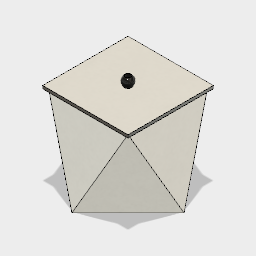
Nagomi v11 (Autodesk Fusion 360 design; units mm, degrees)
Autodesk Fusion 360 part; units mm, degrees
sketch "Sketch1" plane through (0, 0, 0) normal (0, 1, 0) x (1, 0, 0)
  line L0 (40, -40) -> (-40, -40)
  line L1 (-40, -40) -> (-40, 40)
  line L2 (-40, 40) -> (40, 40)
  line L3 (40, 40) -> (40, -40)
  line L4 (40, -40) -> (-40, 40) construction
  line L5 (-40, -40) -> (40, 40) construction
  dimension "d1" = 80
  dimension "d2" = 80
  measures "d1" distance of L1.end L2.end
  measures "d2" distance of L0.end L1.end
extrude "Extrude1" add sketch "Sketch1" along normal blind 80 draft 11.7 makes body 1
ref_plane "WorkPlane1" through (0, 80, 0) normal (0, 1, 0) x (1, 0, 0)
mirror "Mirror1" about plane through (0, 80, 0) normal (0, 1, 0) of bodies 1 makes body 2
move_body "Move1" bodies 2 to x (0.707107, 0, -0.707107) y (0, 1, 0) z (0.707107, 0, 0.707107) at (0, 0, 0)
move_body "Move2" bodies 2 to x (1, 0, 0) y (0, 1, 0) z (0, 0, 1) at (0, -80, 0)
combine "Combine1" operation intersect target body 1 tool bodies 2
shell "Shell1" thickness 2 removed faces 1 at (-18.8557, 80, 0.0004) on bodies 1
move_body "Move3" bodies 1 to x (0.707107, 0, -0.707107) y (0, 1, 0) z (0.707107, 0, 0.707107) at (0, 0, 0)
ref_plane "WorkPlane3" through (0, 75.2, 0) normal (0, 1, 0) x (0.707107, 0, -0.707107)
sketch "Sketch5" plane through (0, 75.2, 0) normal (0, 1, 0) x (1, 0, 0)
  line L0 (-37.9576, 37.9576) -> (37.9576, 37.9576)
  line L1 (37.9576, 37.9576) -> (37.9576, -37.9576)
  line L2 (37.9576, -37.9576) -> (-37.9576, -37.9576)
  line L3 (-37.9576, -37.9576) -> (-37.9576, 37.9576)
  point P0 (-37.9576, 37.9576)
  point P1 (37.9576, -37.9576)
extrude "Extrude2" add sketch "Sketch5" along normal blind 4.8 separate body makes body 3
ref_plane "WorkPlane4" through (0, 80, 0) normal (0, 1, 0) x (0, 0, 1)
sketch "Sketch6" plane through (0, 80, 0) normal (0, 1, 0) x (1, 0, 0)
  line L0 (-40, -39.9981) -> (-40, 39.9981)
  line L1 (-40, -37.8323) -> (-43, -37.8323) construction
  line L2 (39.9981, -40) -> (-39.9981, -40)
  line L3 (-36.5496, -40) -> (-36.5496, -43) construction
  line L4 (-36.5496, -43) -> (-44, -43)
  line L5 (-43, -37.8323) -> (-43, -43)
  line L6 (-39.9981, 40) -> (39.9981, 40)
  line L7 (35.8022, 40) -> (35.8022, 43) construction
  line L8 (40, 39.9981) -> (40, -39.9981)
  line L9 (40, 37.0082) -> (43, 37.0082) construction
  line L10 (43, 37.0082) -> (43, 45)
  line L11 (35.8022, 43) -> (43, 43)
  line L12 (43, 43) -> (-43, 43)
  line L13 (-43, 43) -> (-43, -43)
  line L14 (-43, -43) -> (43, -43)
  line L15 (43, -43) -> (43, 43)
  dimension "d18" = 3
  dimension "d19" = 3
  dimension "d20" = 3
  dimension "d21" = 3
  measures "d18" distance of L1.start L1.end
  measures "d19" distance of L3.start L3.end
  measures "d20" distance of L7.start L7.end
  measures "d21" distance of L9.start L9.end
extrude "Extrude3" add sketch "Sketch6" along normal blind 3 contours L0 L2 L6 L8 | L4 L5 L10 L11 L12 L13 L14 L15 bodies 3
sphere "SpherePrimitive1" add diameter 11 placed x (-1, 0, 0) y (0, 0, 1) z (0, 1, 0) at (0, 83, 0) separate body makes body 4
move_body "Move4" bodies 4 to x (1, 0, 0) y (0, 1, 0) z (0, 0, 1) at (0, 4, 0)
combine "Combine2" operation add target body 3 tool bodies 4
sketch "Sketch8" plane through (0, 83, 0) normal (0, 1, 0) x (-1, 0, 0)
  circle A0 centre (0, 0) radius 3.7749
  line L0 (-43, 43) -> (-43, -43)
  line L1 (-43, -43) -> (43, -43)
  line L2 (43, -43) -> (43, 43)
  line L3 (43, 43) -> (-43, 43)
ref_plane "WorkPlane5" through (0, 93, 0) normal (0, 1, 0) x (-1, 0, 0)
sketch "Sketch9" plane through (0, 93, 0) normal (0, 1, 0) x (1, 0, 0)
  circle A0 centre (0, 0) radius 2.5
  dimension "d29" = 5
  measures "d29" diameter of A0
extrude "Extrude4" cut sketch "Sketch9" against normal up to surface (17.8 mm away) bodies 3
fillet "Fillet1" radius 0.25 1 edges at (-2.3308, 91.899, -0.904) on bodies 3
copy_body "Body->Comp1" bodies 3 removing the originals makes body 5 in component "lead"
copy_body "Body->Comp2" bodies 1 removing the originals makes body 6 in component "triangle box"
component "lead" placed x (1, 0, 0) y (0, 1, 0) z (0, 0, 1) at (0, 0, 0)
component "triangle box" placed x (1, 0, 0) y (0, 1, 0) z (0, 0, 1) at (0, 0, 0)
named bodies: "triangle box", "lead"
